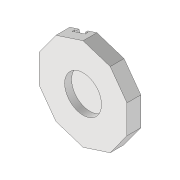
# Autodesk Inventor part: Unterteil
Saved by Autodesk Inventor 2020 (Build 240168000, 168)
## iProperties
Created: 2020-03-18
Part Number: Unterteil
Material: Generisch
Document SubType Name: Modeling
Designer: franz
Density: 1 g/cm^3
Appearance: Vorgabe
Author: franz
Autodesk Inventor part; units mm, degrees
ref_plane "YZ Plane" through (0, 0, 0) normal (1, 0, 0) x (0, 1, 0)
ref_plane "XZ Plane" through (0, 0, 0) normal (0, 1, 0) x (-1, 0, 0)
ref_plane "XY Plane" through (0, 0, 0) normal (0, 0, 1) x (1, 0, 0)
sketch "Skizze1" plane through (0, 0, 0) normal (0, 0, 1) x (1, 0, 0)
  circle A0 centre (0, 0) radius 40
  line L0 (0, 100) -> (58.7785, 80.9017)
  line L1 (58.7785, 80.9017) -> (95.1057, 30.9017)
  line L2 (95.1057, 30.9017) -> (95.1057, -30.9017)
  line L3 (95.1057, -30.9017) -> (58.7785, -80.9017)
  line L4 (58.7785, -80.9017) -> (0, -100)
  line L5 (0, -100) -> (-58.7785, -80.9017)
  line L6 (-58.7785, -80.9017) -> (-95.1057, -30.9017)
  line L7 (-95.1057, -30.9017) -> (-95.1057, 30.9017)
  line L8 (-95.1057, 30.9017) -> (-58.7785, 80.9017)
  line L9 (-58.7785, 80.9017) -> (0, 100)
  dimension "d0" = 80
  dimension "d1" = 100
  constraints: 20 end point, 2 coincident, 1 centre point, 21 other
  measures "d0" diameter of A0
  measures "d1" distance of point (0, 0) L0.start
extrude "Extrusion1" add sketch "Skizze1" along normal blind 15
sketch "Skizze3" plane through (0, 0, 0) normal (0, 0, -1) x (-1, 0, 0)
  line L0 (-95.1057, -30.9017) -> (-95.1057, 30.9017) projected
  line L1 (-58.7785, -80.9017) -> (-95.1057, -30.9017) projected
  line L2 (0, -100) -> (-58.7785, -80.9017) projected
  line L3 (58.7785, -80.9017) -> (0, -100) projected
  line L4 (95.1057, -30.9017) -> (58.7785, -80.9017) projected
  line L5 (95.1057, 30.9017) -> (95.1057, -30.9017) projected
  line L6 (58.7785, 80.9017) -> (95.1057, 30.9017) projected
  line L7 (0, 100) -> (58.7785, 80.9017) projected
  line L8 (-58.7785, 80.9017) -> (0, 100) projected
  line L9 (-95.1057, 30.9017) -> (-58.7785, 80.9017) projected
  circle A0 centre (0, 0) radius 40 projected
extrude "Extrusion2" add sketch "Skizze3" along normal blind 15 contours L0 L9 L8 L7 L6 L5 L4 L3 L2 L1 | A0
sketch "Skizze4" plane through (-58.7785, 80.9017, 15) normal (-0.309, 0.9511, 0) x (0.9511, 0.309, 0)
  line L0 (61.8034, 30) -> (0, 30) projected
  line L1 (40.9017, 30) -> (40.9017, 25)
  line L2 (40.9017, 25) -> (45.9017, 25)
  line L3 (45.9017, 25) -> (45.9017, 20)
  line L4 (45.9017, 20) -> (15.9017, 20)
  line L5 (15.9017, 20) -> (15.9017, 25)
  line L6 (15.9017, 25) -> (20.9017, 25)
  line L7 (20.9017, 25) -> (20.9017, 30)
  point P0 (30.9017, 15)
  dimension "d6" = 20
  dimension "d7" = 10
  dimension "d8" = 30
  dimension "d9" = 15
  dimension "d10" = 5
  dimension "d11" = 5
  constraints: 14 end point, 5 perpendicular, 4 point on line, 1 vertical
  measures "d6" distance between parallel lines of L7 L1
  measures "d7" distance from line of L1 point (30.902, 15)
  measures "d8" distance between parallel lines of L5 L3
  measures "d9" distance from line of point (30.902, 15) L3
  measures "d10" distance of L1.start L1.end
  measures "d11" distance of L2.end L3.end
extrude "Extrusion3" cut sketch "Skizze4" against normal through all
equation "\"d7\" = 0.5 * d6"
equation "\"d9\" = 0.5 * d8"
